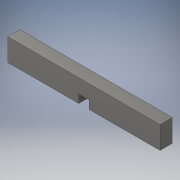
# Autodesk Inventor part: VS-009 (SLIDE KEY)
Saved by Autodesk Inventor 2017 SP1 (Build 210196100, 196)
## iProperties
Created: 2016-12-07
Part Number: VS-009 (SLIDE KEY)
Material: Steel, Carbon
Document SubType Name: Modeling
Designer: OCCC
Density: 7.85 g/cm^3
Appearance: Semi-Polished
Author: OCCC
Autodesk Inventor part; units mm, degrees
ref_plane "YZ Plane" through (0, 0, 0) normal (1, 0, 0) x (0, 1, 0)
ref_plane "XZ Plane" through (0, 0, 0) normal (0, 1, 0) x (-1, 0, 0)
ref_plane "XY Plane" through (0, 0, 0) normal (0, 0, 1) x (1, 0, 0)
sketch "Sketch1" plane through (0, 0, 0) normal (0, 0, 1) x (1, 0, 0)
  line L0 (0, 0) -> (0, 8.6487)
  line L1 (0, 8.6487) -> (58.7375, 8.6487)
  line L2 (58.7375, 8.6487) -> (58.7375, 0)
  line L3 (58.7375, 0) -> (31.3531, 0)
  line L4 (31.3531, 0) -> (31.3531, 3.175)
  line L5 (31.3531, 3.175) -> (27.3844, 3.175)
  line L6 (27.3844, 3.175) -> (27.3844, 0)
  line L7 (27.3844, 0) -> (0, 0)
  dimension "d0" = 3.9688
  dimension "d1" = 3.175
  dimension "d2" = 58.7375
  dimension "d3" = 8.6487
  constraints: 16 end point, 7 perpendicular, 1 collinear, 1 point on line, 1 vertical
  measures "d0" distance between parallel lines of L4 L6
  measures "d1" distance between parallel lines of L3 L5
  measures "d2" distance of L0.end L1.end
  measures "d3" distance between parallel lines of L7 L1
extrude "Extrusion1" add sketch "Sketch1" against normal blind 4.7117
body "Solid1"
